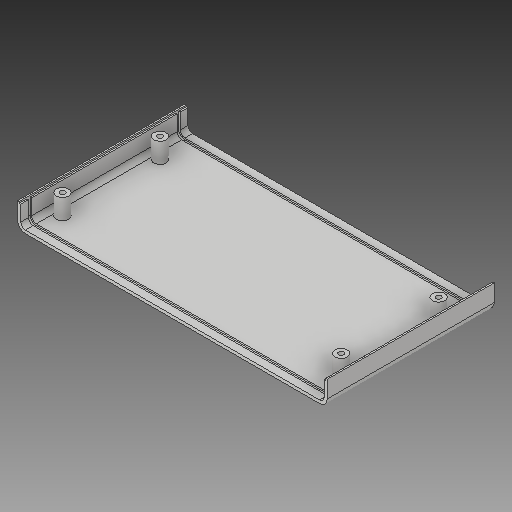
# Autodesk Inventor part: case-bottom
Saved by Autodesk Inventor 2017 (Build 210142000, 142)
## iProperties
Created: 2020-10-01
Part Number: case-bottom
Material: Generic
Document SubType Name: Modeling
Designer: jferner
Density: 1 g/cm^3
Appearance: Default
fillet2: 5.000 mm
thickness2: 2.000 mm
caseBottomWidth2: 200.000 mm
caseBottomHeight2: 16.000 mm
caseBottomDepth2: 108.000 mm
frontBackOffset2: -5.000 mm
filletInner2: 3.000 mm
filletMid2: 4.000 mm
Author: jferner
Autodesk Inventor part; units mm, degrees
ref_plane "YZ Plane" through (0, 0, 0) normal (1, 0, 0) x (0, 1, 0)
sketch "Sketch1" plane through (0, 0, 0) normal (0, 0, 1) x (1, 0, 0)
  line L0 (0, 16) -> (0, 5)
  line L1 (5, 0) -> (195, 0)
  line L2 (200, 5) -> (200, 16)
  arc A0 (0, 5) -> (5, 0) centre (5, 5) ccw
  arc A1 (195, 0) -> (200, 5) centre (195, 5) ccw
  line L3 (2, 16) -> (2, 5)
  arc A2 (2, 5) -> (5, 2) centre (5, 5) ccw
  line L4 (5, 2) -> (195, 2)
  arc A3 (195, 2) -> (198, 5) centre (195, 5) ccw
  line L5 (198, 5) -> (198, 16)
  line L6 (0, 16) -> (2, 16)
  line L7 (198, 16) -> (200, 16)
  point P0 (0, 0)
  dimension "fillet2" = 5
  dimension "thickness2" = 2
  dimension "caseBottomWidth2" = 200
  dimension "caseBottomHeight2" = 16
  constraints: 16 end point, 8 point on circle, 4 centre point, 4 perpendicular, 4 tangent, 2 collinear, 2 point on line, 1 equal radius, 1 horizontal, 1 vertical, 4 other
  measures "fillet2" radius of A0
  measures "thickness2" distance between parallel lines of L0 L3
  measures "caseBottomWidth2" distance between parallel lines of L2 L0
  measures "caseBottomHeight2" distance between parallel lines of L6 L1
extrude "Extrusion1" add sketch "Sketch1" along normal blind 108
ref_plane "Work Plane1" through (0, 0, 103) normal (0, 0, 1) x (1, 0, 0)
sketch "Sketch3" plane through (0, 0, 103) normal (0, 0, 1) x (1, 0, 0)
  line L0 (2, 16) -> (1, 16)
  line L1 (2, 16) -> (2, 5)
  line L2 (1, 16) -> (1, 5)
  line L3 (195, 2) -> (5, 2) projected
  line L4 (195, 2) -> (5, 2)
  line L5 (198, 16) -> (198, 5) projected
  line L6 (198, 16) -> (198, 5)
  line L7 (198, 16) -> (199, 16)
  line L8 (199, 16) -> (199, 5)
  line L9 (5, 1) -> (195, 1)
  arc A0 (2, 5) -> (5, 2) centre (5, 5) ccw
  arc A1 (195, 2) -> (198, 5) centre (195, 5) ccw
  arc A2 (1, 5) -> (5, 1) centre (5, 5) ccw
  arc A3 (195, 1) -> (199, 5) centre (195, 5) ccw
  point P0 (0, 0)
  dimension "d8" = 1
  dimension "d9" = 1
  dimension "d10" = 1
  dimension "filletInner2" = 3
  dimension "filletMid2" = 4
  constraints: 16 end point, 8 point on circle, 8 tangent, 4 centre point, 4 horizontal, 3 vertical, 2 equal radius, 1 collinear, 1 parallel
  measures "d8" distance of L0.start L0.end
  measures "d9" distance of L5.start L7.end
  measures "d10" distance between parallel lines of L9 L4
  measures "filletInner2" radius of A0
  measures "filletMid2" radius of A2
extrude "Extrusion2" cut sketch "Sketch3" against normal blind 2
ref_plane "Work Plane2" through (0, 0, 5) normal (0, 0, -1) x (-1, 0, 0)
sketch "Sketch5" plane through (0, 0, 5) normal (0, 0, -1) x (-1, 0, 0)
  line L0 (-200, 16) -> (-198, 16) projected
  line L1 (-198, 16) -> (-198, 5)
  line L2 (-199, 16) -> (-199, 5)
  line L3 (-2, 5) -> (-2, 16) projected
  line L4 (-2, 16) -> (-2, 5)
  line L5 (-2, 16) -> (0, 16) projected
  line L6 (-1, 16) -> (-1, 5)
  line L7 (-195, 2) -> (-5, 2)
  line L8 (-195, 1) -> (-5, 1)
  line L9 (-195, 2) -> (-5, 2) projected
  arc A0 (-198, 5) -> (-195, 2) centre (-195, 5) ccw
  arc A1 (-5, 2) -> (-2, 5) centre (-5, 5) ccw
  arc A2 (-199, 5) -> (-195, 1) centre (-195, 5) ccw
  arc A3 (-5, 1) -> (-1, 5) centre (-5, 5) ccw
  point P0 (0, 0)
  dimension "d21" = 1
  dimension "d22" = 3
  dimension "d23" = 4
  constraints: 12 end point, 8 point on circle, 8 tangent, 4 centre point, 4 vertical, 2 equal radius, 2 horizontal, 2 midpoint, 1 collinear
  measures "d21" distance between parallel lines of L7 L8
  measures "d22" radius of A0
  measures "d23" radius of A2
extrude "Extrusion4" cut sketch "Sketch5" against normal blind 2
sketch "Sketch7" plane through (0, 0, 108) normal (0, 0, 1) x (1, 0, 0)
  line L0 (2, 16) -> (0, 16) projected
  line L1 (2, 16) -> (1, 16)
  line L2 (1, 16) -> (1, 15)
  line L3 (1, 15) -> (2, 15)
  line L4 (2, 15) -> (2, 16)
  line L5 (199, 5) -> (199, 16) projected
  line L6 (198, 16) -> (198, 5) projected
  line L7 (199, 16) -> (198, 16)
  line L8 (198, 16) -> (198, 15)
  line L9 (198, 15) -> (199, 15)
  line L10 (199, 15) -> (199, 16)
  point P0 (0, 0)
  dimension "d28" = 1
  dimension "d29" = 1
  constraints: 16 end point, 4 parallel, 2 horizontal, 2 perpendicular, 1 collinear, 1 point on line
  measures "d28" distance between parallel lines of L0 L3
  measures "d29" distance between parallel lines of L4 L2
extrude "Extrusion6" cut sketch "Sketch7" against normal through all
sketch "Sketch8" plane through (5, 2, 101) normal (0, 1, 0) x (1, 0, 0)
  circle A0 centre (4, 76) radius 4
  line L0 (-5, 101) -> (-5, -7) projected
  line L1 (190, 101) -> (0, 101) projected
  circle A1 centre (184, 76) radius 4
  circle A2 centre (4, 13) radius 4
  circle A3 centre (184, 13) radius 4
  dimension "d32" = 9
  dimension "d33" = 25
  dimension "d34" = 8
  dimension "d37" = 180
  dimension "d40" = 63
  constraints: 4 centre point, 1 horizontal, 1 vertical, 6 other
  measures "d32" distance from line of L0 A0.centre
  measures "d33" distance from line of L1 A0.centre
  measures "d34" diameter of A0
  measures "d37" distance of A0.centre A1.centre
  measures "d40" distance of A0.centre A2.centre
extrude "Extrusion7" add sketch "Sketch8" along normal blind 13
sketch "Sketch9" plane through (9, 15, 88) normal (0, 1, 0) x (1, 0, 0)
  circle A0 centre (0, 63) radius 4 projected
  circle A1 centre (0, 63) radius 1.7
  circle A2 centre (0, 0) radius 1.7
  circle A3 centre (180, 0) radius 1.7
  circle A4 centre (180, 63) radius 4 projected
  circle A5 centre (180, 63) radius 1.7
  circle A6 centre (180, 0) radius 4 projected
  circle A7 centre (0, 0) radius 4 projected
  point P0 (-9, 88)
  dimension "d45" = 3.4
  constraints: 4 centre point, 3 equal radius, 2 coincident, 2 concentric
  measures "d45" diameter of A1
extrude "Extrusion8" cut sketch "Sketch9" against normal blind 12 contours A1 | A2 | A3 | A5
equation "\"fillet2\" = fillet"
equation "\"thickness2\" = thickness"
equation "\"caseBottomWidth2\" = caseBottomWidth"
equation "\"caseBottomHeight2\" = caseBottomHeight"
equation "\"caseBottomDepth2\" = caseBottomDepth"
equation "\"d8\" = 0.5 * thickness2"
equation "\"d9\" = 0.5 * thickness2"
equation "\"d10\" = 0.5 * thickness2"
equation "\"filletInner2\" = filletInner"
equation "\"filletMid2\" = filletMid"
equation "\"d13\" = thickness2"
equation "\"d21\" = 0.5 * thickness2"
equation "\"d22\" = filletInner2"
equation "\"d23\" = filletMid2"
equation "\"d24\" = thickness2"
equation "\"d28\" = lipHeight"
equation "\"d29\" = 0.5 * thickness"
equation "\"d32\" = caseJoinOffsetFromSide"
equation "\"d33\" = caseJoinOffsetFromBack"
equation "\"d34\" = caseJoinDiameter"
equation "\"d37\" = caseJoinSpacingLeftRight"
equation "\"d40\" = caseJoinSpacingFrontBack"
equation "\"d43\" = caseBottomHeight2 - 1.5 * thickness"
equation "\"d45\" = holeDiameter"
equation "\"d46\" = caseBottomHeight2 - 2 * thickness"
equation "\"frontBackOffset2\" = frontBackOffset"
equation "\"d15\" = frontBackOffset2"
equation "\"fillet\" = 5"
equation "\"thickness\" = 2"
equation "\"caseBottomWidth\" = 200"
equation "\"caseBottomHeight\" = 16"
equation "\"caseBottomDepth\" = 108"
equation "\"filletInner\" = 3"
equation "\"filletMid\" = 4"
equation "\"lipHeight\" = 1"
equation "\"caseJoinOffsetFromSide\" = 9"
equation "\"caseJoinOffsetFromBack\" = 25"
equation "\"caseJoinDiameter\" = 8"
equation "\"caseJoinSpacingLeftRight\" = 180"
equation "\"caseJoinSpacingFrontBack\" = 63"
equation "\"holeDiameter\" = 3.4"
equation "\"frontBackOffset\" = -5"
body "Solid1"
